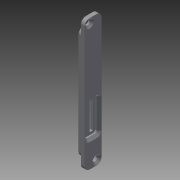
# Autodesk Inventor part: IOModulePlate02
Saved by Autodesk Inventor 2013 (Build 170138000, 138)
## iProperties
Created: 2014-07-14
Part Number: IOModulePlate02
Material: Generic
Document SubType Name: Modeling
Designer: spichelh
Density: 1 g/cm^3
Author: spichelh
Autodesk Inventor part; units mm, degrees
ref_plane "YZ Plane" through (0, 0, 0) normal (1, 0, 0) x (0, 1, 0)
ref_plane "XZ Plane" through (0, 0, 0) normal (0, 1, 0) x (-1, 0, 0)
ref_plane "XY Plane" through (0, 0, 0) normal (0, 0, 1) x (1, 0, 0)
sketch "Sketch1" plane through (0, 0, 0) normal (1, 0, 0) x (0, 1, 0)
  line L0 (2, 0) -> (50.8, 0)
  line L1 (52.8, -2) -> (52.8, -4.8)
  line L2 (50.8, -6.8) -> (2, -6.8)
  line L3 (0, -4.8) -> (0, -2)
  arc A0 (2, 0) -> (0, -2) centre (2, -2) ccw
  arc A1 (0, -4.8) -> (2, -6.8) centre (2, -4.8) ccw
  arc A2 (50.8, -6.8) -> (52.8, -4.8) centre (50.8, -4.8) ccw
  arc A3 (52.8, -2) -> (50.8, 0) centre (50.8, -2) ccw
  line L4 (26.4, 0) -> (26.4, -6.5481) construction
  line L5 (52.8, -3.4) -> (39.7965, -3.4) construction
  circle A4 centre (1.9, -1.9) radius 1 construction
  circle A5 centre (50.9, -1.9) radius 1
  circle A6 centre (50.9, -4.9) radius 1 construction
  circle A7 centre (1.9, -4.9) radius 1
  point P0 (0, 0)
  point P1 (52.8, 0)
  point P2 (0, -6.8)
  dimension "d0" = 52.8
  dimension "d1" = 6.8
  dimension "d2" = 2
  dimension "d35" = 2
  dimension "d36" = 0.1
  dimension "d37" = 0.1
  constraints: 12 end point, 8 centre point, 8 point on circle, 8 tangent, 6 point on line, 3 equal radius, 3 parallel, 3 symmetric about line, 2 midpoint, 2 perpendicular, 1 horizontal, 3 other
  measures "d0" distance of point (0, 0) point (52.8, 0)
  measures "d1" distance of point (0, -6.8) point (0, 0)
  measures "d2" radius of A0
  measures "d35" diameter of A4
  measures "d36" horizontal distance of A4.centre A0.centre
  measures "d37" horizontal distance of A4.centre A0.centre
extrude "Extrusion1" add sketch "Sketch1" along normal blind 1.5
chamfer "Chamfer1" distance 0.8 angle 45 2 edges at (1.5, 49.9, -1.9) (1.5, 0.9, -4.9)
sketch "Sketch2" plane through (1.5, 0, 0) normal (1, 0, 0) x (0, 0, -1)
  line L0 (0, 50.8) -> (0, 2) projected
  line L1 (2, 23.5) -> (4.8, 23.5)
  line L2 (5.8, 22.5) -> (5.8, 11.5)
  line L3 (4.8, 10.5) -> (2, 10.5)
  line L4 (1, 11.5) -> (1, 22.5)
  arc A0 (5.8, 22.5) -> (4.8, 23.5) centre (4.8, 22.5) ccw
  arc A1 (4.8, 10.5) -> (5.8, 11.5) centre (4.8, 11.5) ccw
  arc A2 (1, 11.5) -> (2, 10.5) centre (2, 11.5) ccw
  arc A3 (2, 23.5) -> (1, 22.5) centre (2, 22.5) ccw
  line L5 (6.8, 2) -> (6.8, 50.8) projected
  line L6 (2, 0) -> (4.8, 0) projected
  point P0 (0, 0)
  dimension "d11" = 1
  dimension "d19" = 1
  dimension "d20" = 13
  dimension "d21" = 1
  dimension "d22" = 1
  dimension "d23" = 1
  dimension "d24" = 1
  dimension "d25" = 10.5
  constraints: 8 end point, 8 point on circle, 8 tangent, 4 centre point, 2 parallel, 1 horizontal, 1 perpendicular
  measures "d11" distance between parallel lines of L0 L4
  measures "d19" distance between parallel lines of L5 L2
  measures "d20" distance between parallel lines of L3 L1
  measures "d21" radius of A0
  measures "d22" radius of A3
  measures "d23" radius of A1
  measures "d24" radius of A2
  measures "d25" distance between parallel lines of L6 L3
extrude "Extrusion2" cut sketch "Sketch2" against normal blind 1.5
sketch "Sketch3" plane through (0, 0, 0) normal (-1, 0, 0) x (0, 0, 1)
  arc A0 (-4.8, 23.5) -> (-5.8, 22.5) centre (-4.8, 22.5) ccw projected
  arc A1 (-1, 22.5) -> (-2, 23.5) centre (-2, 22.5) ccw projected
  line L0 (-1, 22.5) -> (-1, 11.5) projected
  line L1 (-2, 10.5) -> (-4.8, 10.5) projected
  arc A2 (-5.8, 11.5) -> (-4.8, 10.5) centre (-4.8, 11.5) ccw projected
  line L2 (-5.8, 11.5) -> (-5.8, 22.5) projected
  line L3 (0, 50.8) -> (0, 2) projected
  line L4 (-4.8, 52.8) -> (-2, 52.8) projected
  line L5 (-4.8, 48.8) -> (-2, 48.8)
  line L6 (0, 46.8) -> (0, 6)
  line L7 (-2, 4) -> (-4.8, 4)
  line L8 (-6.8, 6) -> (-6.8, 46.8)
  arc A3 (-4.8, 48.8) -> (-6.8, 46.8) centre (-4.8, 46.8) ccw
  arc A4 (0, 46.8) -> (-2, 48.8) centre (-2, 46.8) ccw
  arc A5 (-2, 4) -> (0, 6) centre (-2, 6) ccw
  arc A6 (-6.8, 6) -> (-4.8, 4) centre (-4.8, 6) ccw
  line L9 (-3.4, 52.8) -> (-3.4, 49.069) construction
  line L10 (0, 26.4) -> (-3, 26.4) construction
  line L11 (-6.8, 26.4) -> (-12.1303, 26.4) construction
  line L12 (-4.8, 23.5) -> (-4.8, 23.5)
  line L13 (-5.8, 22.5) -> (-5.8, 11.5)
  line L14 (-4.8, 10.5) -> (-4.8, 10.5)
  line L15 (-4.8, 10.5) -> (-4.8, 23.5)
  line L16 (-3.5, 23.5) -> (-2, 23.5)
  line L17 (-1, 22.5) -> (-1, 11.5)
  line L18 (-2, 10.5) -> (-3.5, 10.5)
  line L19 (-3.5, 10.5) -> (-3.5, 23.5)
  arc A7 (-4.8, 23.5) -> (-5.8, 22.5) centre (-4.8, 22.5) ccw
  arc A8 (-5.8, 11.5) -> (-4.8, 10.5) centre (-4.8, 11.5) ccw
  arc A9 (-1, 22.5) -> (-2, 23.5) centre (-2, 22.5) ccw
  arc A10 (-2, 10.5) -> (-1, 11.5) centre (-2, 11.5) ccw
  line L20 (-4.8, 23.5) -> (-2, 23.5) projected
  line L21 (-4.8, 22.5) -> (-3.5, 22.5)
  line L22 (-4.8, 11.5) -> (-3.5, 11.5)
  point P0 (0, 0)
  point P1 (0, 4)
  point P2 (0, 48.8)
  point P3 (-6.8, 4)
  point P4 (-6.8, 45.8508)
  point P5 (-6.8, 31.9198)
  point P6 (-6.8, 26.4798)
  point P7 (-6.8, 11.7389)
  dimension "d14" = 6.8
  dimension "d15" = 44.8
  dimension "d16" = 2
  dimension "d29" = 1
  dimension "d30" = 2.5
  dimension "d31" = 1
  dimension "d32" = 1.3
  dimension "d33" = 1
  dimension "d34" = 1
  constraints: 34 end point, 16 point on circle, 16 tangent, 10 point on line, 8 centre point, 7 perpendicular, 6 equal radius, 6 parallel, 3 horizontal, 3 midpoint, 2 collinear, 1 other
  measures "d14" distance of point (0, 4) point (-6.8, 4)
  measures "d15" distance of point (0, 48.8) point (0, 4)
  measures "d16" radius of A3
  measures "d29" radius of A7
  measures "d30" distance between parallel lines of L0 L19
  measures "d31" distance between parallel lines of L2 L15
  measures "d32" distance between parallel lines of L19 L15
  measures "d33" distance between parallel lines of L20 L21
  measures "d34" distance between parallel lines of L22 L1
extrude "Extrusion3" add sketch "Sketch3" along normal blind 1 contours L15 A2 L2 A0 | L20 L19 L21 L15 | L16 A1 L0 A10 L1 L19 | L22 L19 L1 L15 | L3 A5 L7 A6 L8 A3 L5 A4
chamfer "Chamfer2" distance 1 angle 45 8 edges at (1.5, 17, -5.8) (1.5, 10.7929, -5.5071) (1.5, 10.5, -3.4) (1.5, 10.7929, -1.2929) (1.5, 17, -1) (1.5, 23.2071, -1.2929) (1.5, 23.5, -3.4) (1.5, 23.2071, -5.5071)
body "Solid1"
